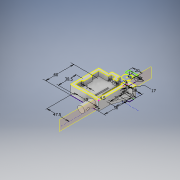
# Autodesk Inventor part: Housing
Saved by Autodesk Inventor 2017 (Build 210142000, 142)
## iProperties
Created: 2018-10-15
Part Number: Housing
Material: Generic
Document SubType Name: Modeling
Designer: Tom
Density: 1 g/cm^3
Appearance: Default
Author: Tom
Autodesk Inventor part; units mm, degrees
ref_plane "XZ Plane" through (0, 0, 0) normal (0, 1, 0) x (-1, 0, 0)
ref_plane "XY Plane" through (0, 0, 0) normal (0, 0, 1) x (1, 0, 0)
sketch "Sketch1" plane through (0, 0, 0) normal (0, 1, 0) x (-1, 0, 0)
  line L0 (0, 0) -> (0, -60)
  line L1 (0, 0) -> (-50, 0)
  line L2 (-5, -60) -> (-5, -5)
  line L3 (-5, -5) -> (-50, -5)
  line L4 (-47.5, 69.0442) -> (-47.5, -71.5611) construction
  line L5 (-50, 0) -> (-55, 0)
  line L6 (-55, 0) -> (-55, -50)
  line L7 (-55, -50) -> (-75, -50)
  line L8 (-75, -50) -> (-75, -60)
  line L9 (-75, -60) -> (-45, -60)
  line L10 (-5, -60) -> (-21, -60)
  circle A0 centre (-47.5, -73.124) radius 8.5
  line L11 (16.7028, -43.5) -> (-102.7124, -43.5) construction
  line L12 (-45, -26.5) -> (-50, -26.5)
  line L13 (-50, -26.5) -> (-50, -60.5)
  line L14 (-50, -60.5) -> (-45, -60.5)
  line L15 (-45, -60.5) -> (-45, -26.5)
  line L16 (-45, -43.5) -> (-50, -43.5) construction
  line L17 (-21, -60) -> (-21, -67.124)
  line L18 (-21, -67.124) -> (-30, -67.124)
  line L19 (-39, -67.124) -> (-39, -60)
  line L20 (-39, -60) -> (-45, -60) construction
  line L21 (-15.952, -100.4576) -> (-35.952, -100.4576)
  line L22 (-35.952, -108.4576) -> (-15.952, -108.4576)
  line L23 (-15.952, -108.4576) -> (-15.952, -100.4576)
  line L24 (-15.952, -73.124) -> (-76.4965, -73.124) construction
  line L25 (-30, -57.9879) -> (-30, -83.8601) construction
  line L26 (-25.952, -100.4576) -> (-25.952, -108.4576) construction
  line L27 (-45, -31) -> (-50, -31) construction
  line L28 (-50, -31) -> (-50, -56)
  line L29 (-50, -56) -> (-45, -56) construction
  line L30 (-45, -56) -> (-45, -31)
  line L31 (-45, -56) -> (-50, -56)
  line L32 (-45, -65.1391) -> (-45, -56)
  line L33 (-45, -56) -> (-50, -56)
  line L34 (-50, -56) -> (-50, -65)
  line L35 (-50, -65) -> (-45, -65)
  line L36 (-45, -65) -> (-45, -56)
  arc A1 (-35.952, -108.4576) -> (-35.952, -100.4576) centre (-43.452, -104.4576) ccw
  line L37 (-30, -67.124) -> (-39, -67.124)
  point P0 (-47.5, -43.5)
  point P1 (-30, -73.124)
  dimension "d9" = 17
  dimension "d0" = 60
  dimension "d1" = 50
  dimension "d2" = 5
  dimension "d3" = 47.5
  dimension "d4" = 5
  dimension "d5" = 50
  dimension "d6" = 20
  dimension "d7" = 30
  dimension "d10" = 38.5
  dimension "d11" = 5
  dimension "d12" = 34
  dimension "d13" = 20
  dimension "d14" = 8
  dimension "d57" = 25
  dimension "d58" = 4.5
  dimension "d59" = 5
  dimension "d60" = 9
  dimension "d61" = 17
  dimension "d62" = 9
  dimension "d63" = 9
  dimension "d64" = 9
  dimension "d65" = 6
  constraints: 76 end point, 11 horizontal, 10 perpendicular, 9 point on line, 7 parallel, 5 midpoint, 5 vertical, 2 collinear, 2 point on circle, 1 centre point, 4 other
  measures "d0" distance of L0.start L0.end
  measures "d1" distance of L0.start L1.end
  measures "d2" distance between parallel lines of L0 L2
  measures "d3" distance between parallel lines of L4 L0
  measures "d4" distance of L1.end L5.end
  measures "d5" distance of L5.end L6.end
  measures "d6" distance of L6.end L7.end
  measures "d7" distance of L8.end L9.end
  measures "d10" distance between parallel lines of L3 L11
  measures "d11" distance of L14.end L13.end
  measures "d12" distance of L13.end L12.end
  measures "d13" distance of L22.end L22.start
  measures "d14" distance of L22.start L21.end
  measures "d57" distance of L28.end L27.end
  measures "d58" distance between parallel lines of L12 L27
  measures "d59" distance of L35.end L34.end
  measures "d60" distance of L34.end L33.end
  measures "d61" diameter of A1
  measures "d62" distance edge to line of A1 L26
  measures "d64" distance of L17.end L18.end
  measures "d65" distance between parallel lines of L18 L24
sketch "Sketch2" plane through (0, 0, 0) normal (0, 1, 0) x (-1, 0, 0)
  line L0 (0, 0) -> (-60, 0)
  line L1 (-60, 0) -> (-60, -55)
  line L2 (-57.5, -60) -> (0, -60)
  line L3 (0, -60) -> (0, 0)
  line L4 (-5, -60) -> (-21, -60) projected
  line L5 (-30, -67.124) -> (-39, -67.124) projected
  line L6 (-57.5, -67.124) -> (-72, -67.124)
  line L7 (-72, -67.124) -> (-72, -59.124)
  line L8 (-72, -59.124) -> (-60, -59.124)
  line L9 (-60, -59.124) -> (-60, 0)
  line L10 (-57.5, -67.124) -> (-57.5, -60)
  point P0 (-60, -67.124)
  dimension "d16" = 57.5
  dimension "d73" = 8
  dimension "d76" = 12
  dimension "d77" = 60
  constraints: 18 end point, 3 perpendicular, 2 horizontal, 2 parallel, 2 point on line, 1 collinear
  measures "d16" distance of L2.end L2.start
  measures "d73" distance of L6.end L7.end
  measures "d76" distance between parallel lines of L1 L7
  measures "d77" distance between parallel lines of L3 L1
extrude "Extrusion1" add sketch "Sketch2" along normal blind 20
sketch "Sketch3" plane through (0, 20, 0) normal (0, 1, 0) x (1, 0, 0)
  line L0 (5, 5) -> (55, 5)
  line L1 (55, 5) -> (55, 55)
  line L2 (55, 55) -> (5, 55)
  line L3 (5, 55) -> (5, 5)
  line L4 (0, 0) -> (60, 0) projected
  line L5 (0, 60) -> (0, 0) projected
  dimension "d23" = 5
  dimension "d24" = 5
  dimension "d25" = 50
  dimension "d26" = 50
  constraints: 8 end point, 2 parallel, 1 horizontal, 1 perpendicular
  measures "d23" distance between parallel lines of L5 L3
  measures "d24" distance between parallel lines of L4 L0
  measures "d25" distance of L2.end L0.start
  measures "d26" distance of L1.end L2.end
extrude "Extrusion2" cut sketch "Sketch3" against normal blind 10
sketch "Sketch5" plane through (0, 0, 0) normal (0, -1, 0) x (1, 0, 0)
  line L0 (57.5, -60) -> (0, -60) projected
  line L1 (45, -60.5) -> (45, -26.5) projected
  line L2 (5, -60) -> (5, -5) projected
  line L3 (50, -26.5) -> (50, -60.5) projected
  line L4 (45, -26.5) -> (50, -26.5) projected
  line L5 (50, -60.5) -> (45, -60.5) projected
  line L6 (52, -60) -> (52, -24.5)
  line L7 (52, -24.5) -> (43, -24.5)
  line L8 (43, -24.5) -> (43, -60)
  line L9 (52, -60.5) -> (52, -60)
  line L10 (52, -60) -> (43, -60)
  point P0 (80, -60)
  dimension "d30" = 40
  dimension "d31" = 2
  constraints: 10 end point, 2 point on line, 1 collinear, 1 perpendicular
  measures "d30" distance between parallel lines of L2 L1
  measures "d31" distance between parallel lines of L3 L6
extrude "Extrusion3" cut sketch "Sketch5" against normal through all contours L0 L3 L4 L1 L8 L7 L6 | L0 L1 L4 L3
sketch "Sketch6" plane through (0, 0, 0) normal (0, 0, 1) x (1, 0, 0)
  line L0 (0, 20) -> (60, 20) projected
  line L1 (47.5, 0) -> (47.5, 20) construction
  circle A0 centre (47.5, 10) radius 7
  point P0 (47.5, 0)
  dimension "d34" = 14
  constraints: 2 end point, 1 centre point, 1 coincident, 1 midpoint, 1 perpendicular, 1 point on line
  measures "d34" diameter of A0
extrude "Extrusion4" add sketch "Sketch6" along normal blind 25
ref_plane "Work Plane1" through (54.5, 10, 0) normal (1, 0, 0) x (0, 1, 0)
sketch "Sketch7" plane through (54.5, 10, 0) normal (1, 0, 0) x (0, 1, 0)
  line L0 (7, 25) -> (-7, 25) projected
  line L1 (0, 25) -> (0, 0) construction
  point P0 (-10, 0)
  point P1 (0, 17)
  dimension "d37" = 8
  constraints: 2 end point, 1 midpoint, 1 point on line, 1 vertical
  measures "d37" distance from line of L0 point (0, 17)
hole "Hole1" at (54.5, 10, 17) direction (-1, 0, 0) diameter 5 end through all
sketch "Sketch8" plane through (0, 10, 0) normal (0, 1, 0) x (1, 0, 0)
  line L0 (36, 11.5) -> (39, 11.5)
  line L1 (39, 11.5) -> (39, 43.5)
  line L2 (39, 43.5) -> (36, 43.5)
  line L3 (36, 43.5) -> (36, 11.5)
  line L4 (45, 60.5) -> (45, 26.5) projected
  line L5 (-16.7028, 43.5) -> (102.7124, 43.5) construction
  point P0 (0, 0)
  point P1 (47.5, 43.5)
  dimension "d45" = 6
  dimension "d46" = 32
  dimension "d47" = 3
  constraints: 8 end point, 2 parallel, 1 collinear, 1 horizontal, 1 perpendicular
  measures "d45" distance between parallel lines of L4 L1
  measures "d46" distance of L2.end L0.start
  measures "d47" distance of L0.start L0.end
extrude "Extrusion5" cut sketch "Sketch8" against normal blind 4
sketch "Sketch9" plane through (0, 10, 0) normal (0, 1, 0) x (1, 0, 0)
  line L0 (36, 43.5) -> (39, 43.5) projected
  line L1 (5, 5) -> (5, 55) projected
  line L2 (8, 18.5) -> (5, 18.5)
  line L3 (5, 18.5) -> (5, 38.5)
  line L4 (5, 38.5) -> (8, 38.5)
  line L5 (8, 38.5) -> (8, 18.5)
  point P0 (0, 0)
  dimension "d50" = 3
  dimension "d51" = 5
  dimension "d52" = 20
  constraints: 8 end point, 2 parallel, 1 horizontal, 1 perpendicular, 1 point on line
  measures "d50" distance between parallel lines of L5 L3
  measures "d51" distance between parallel lines of L0 L4
  measures "d52" distance of L4.end L2.start
extrude "Extrusion6" add sketch "Sketch9" along normal up to surface (10 mm away)
fillet "Fillet1" radius 0.6 4 edges at (5, 15, -38.5) (8, 15, -38.5) (8, 15, -18.5) (5, 15, -18.5)
fillet "Fillet2" radius 1 2 edges at (43, 5, -24.5) (52, 5, -24.5)
sketch "Sketch10" plane through (0, 0, 0) normal (0, -1, 0) x (1, 0, 0)
  line L0 (43, -60) -> (0, -60) projected
  line L1 (39, -67.124) -> (39, -60) projected
  line L2 (30, -67.124) -> (39, -67.124) projected
  line L3 (21, -60) -> (21, -67.124) projected
  line L4 (21, -67.124) -> (30, -67.124) projected
  line L5 (39, -60) -> (39, -67.124)
  line L6 (21, -67.124) -> (39, -67.124)
  line L7 (21, -67.124) -> (21, -60)
  point P0 (80, -60)
  constraints: 6 end point, 4 point on line, 2 collinear
extrude "Extrusion7" add sketch "Sketch10" against normal up to surface (20 mm away)
sketch "Sketch11" plane through (0, 20, 0) normal (0, 1, 0) x (1, 0, 0)
  line L0 (39, 67.124) -> (39, 60) projected
  line L1 (21, 67.124) -> (39, 67.124) projected
  line L2 (21, 60) -> (21, 67.124) projected
  line L3 (5, 55) -> (55, 55) projected
  line L4 (25.5, 55) -> (34.5, 55)
  line L5 (34.5, 55) -> (34.5, 61.124)
  line L6 (34.5, 61.124) -> (25.5, 61.124)
  line L7 (25.5, 61.124) -> (25.5, 55)
  dimension "d68" = 6
  dimension "d69" = 4.5
  dimension "d70" = 4.5
  constraints: 8 end point, 2 parallel, 1 horizontal, 1 perpendicular, 1 point on line
  measures "d68" distance between parallel lines of L1 L6
  measures "d69" distance between parallel lines of L2 L7
  measures "d70" distance between parallel lines of L0 L5
extrude "Extrusion8" cut sketch "Sketch11" against normal up to surface (10 mm away)
sketch "Sketch12" plane through (0, 20, 0) normal (0, 1, 0) x (1, 0, 0)
  line L0 (34.5, 61.124) -> (34.5, 55) projected
  line L1 (34.5, 55) -> (43, 55) projected
  line L2 (43, 55) -> (43, 60) projected
  line L3 (43, 60) -> (39, 60) projected
  line L4 (39, 67.124) -> (39, 60) projected
  line L5 (21, 67.124) -> (39, 67.124) projected
  line L6 (21, 60) -> (21, 67.124) projected
  line L7 (21, 60) -> (0, 60) projected
  line L8 (0, 60) -> (0, 0) projected
  line L9 (0, 0) -> (60, 0) projected
  line L10 (60, 0) -> (60, 59.124) projected
  line L11 (60, 59.124) -> (72, 59.124) projected
  line L12 (72, 59.124) -> (72, 67.124) projected
  line L13 (72, 67.124) -> (57.5, 67.124) projected
  line L14 (57.5, 67.124) -> (57.5, 60) projected
  line L15 (57.5, 60) -> (52, 60) projected
  line L16 (52, 60) -> (52, 55) projected
  line L17 (52, 55) -> (55, 55) projected
  line L18 (55, 55) -> (55, 5) projected
  line L19 (55, 5) -> (5, 5) projected
  line L20 (5, 5) -> (5, 17.9) projected
  arc A0 (5.6, 18.5) -> (5, 17.9) centre (5.6, 17.9) ccw projected
  line L21 (7.4, 18.5) -> (5.6, 18.5) projected
  arc A1 (7.4, 18.5) -> (8, 19.1) centre (7.4, 19.1) ccw projected
  line L22 (8, 37.9) -> (8, 19.1) projected
  arc A2 (8, 37.9) -> (7.4, 38.5) centre (7.4, 37.9) ccw projected
  line L23 (5.6, 38.5) -> (7.4, 38.5) projected
  arc A3 (5, 39.1) -> (5.6, 38.5) centre (5.6, 39.1) ccw projected
  line L24 (5, 39.1) -> (5, 55) projected
  line L25 (5, 55) -> (25.5, 55) projected
  line L26 (25.5, 55) -> (25.5, 61.124) projected
  line L27 (25.5, 61.124) -> (34.5, 61.124) projected
  line L28 (65, 73.0401) -> (65, 59.124)
  circle A4 centre (47.5, 73.124) radius 8.5 projected
  point P0 (60, 52.124)
  point P1 (60, 57.124)
  point P2 (62, 59.124)
  dimension "d74" = 9
  constraints: 2 end point, 1 vertical, 2 other
  measures "d74" distance edge to line of A4 L28
sketch "Sketch13" plane through (0, 0, 0) normal (0, -1, 0) x (1, 0, 0)
  line L0 (60, 0) -> (60, -59.124) projected
  line L1 (72, -59.124) -> (60, -24.124)
  line L2 (60, 0) -> (60, -59.124) projected
  line L3 (60, -59.124) -> (60, -24.124)
  line L4 (72, -59.124) -> (60, -59.124)
  dimension "d78" = 35
  constraints: 6 end point, 2 point on line, 1 perpendicular
  measures "d78" distance of L0.end L1.end
extrude "Extrusion9" add sketch "Sketch13" against normal blind 5
equation "\"d70\" = d69"
body "Solid1"
